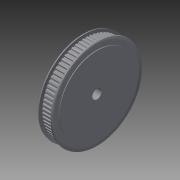
# Autodesk Inventor part: ATP72XL050-A-PUF_a
Saved by Autodesk Inventor 2014 SP2 (Build 180246200, 246)
## iProperties
Created: 2018-08-04
Part Number: ATP72XL050-A-PUF_a
Material: Generic
Catalog Web Link: www.cadenas.de
Description: ATP_ _XL025, ATP_ _XL031, ATP_ _ XL037, ATP_ _XL050, BTP_ _XL025, BTP_ _XL031, BTP_ _XL037, BTP_ _XL050, KTP_ _XL025, KTP_ _XL031, KTP_ _ XL037, KTP_ _XL050, NTP_ _XL025, NTP_ _XL031, NTP_ _ XL037, NTP_ _XL050, MTP_ _XL025, MTP_ _ XL037, MTP_ _XL050, MTPB_ _XL025, MTPB_ _ XL037, MTPB_ _XL050, MTPP_ _XL025, MTPP_ _ XL037, MTPP_ _XL050, STP_ _XL025, STP_ _ XL037, STP_ _XL050_aI-Timing Pulleys XL Type
Vendor: MISUMI
Document SubType Name: Modeling
Designer: psadmin
Manufacturer: MISUMI
Mass: 194.41 g
Surface Area: 364.949 cm^2
Volume: 194.41 cm^3
Density: 1 g/cm^3
Appearance: PSOLRGB-192-192-192
Category: PARTsolutions
Company: MISUMI
Title: ATP72XL050-A-PUF_a
Author: Cadenas PARTsolutions
Comments: Timing Pulleys XL Type
PSOL_IDENT_0: {$CADENAS_DATA\23d-libs\misumi\metric\51_timing_pulleys\timing_pulleys_inch\atp_xl_inch.prj},699 {VT
PSOL_IDENT_1: YP=3D},{NB=ATP72XL050-A-PUF_a},{LINA=ATP72XL050-A-PUF_a},{NN=ATP_ _XL025, ATP_ _XL031, ATP_ _ XL037,
PSOL_IDENT_2: ATP_ _XL050, BTP_ _XL025, BTP_ _XL031, BTP_ _XL037, BTP_ _XL050, KTP_ _XL025, KTP_ _XL031, KTP_ _ X
PSOL_IDENT_3: L037, KTP_ _XL050, NTP_ _XL025, NTP_ _XL031, NTP_ _ XL037, NTP_ _XL050, MTP_ _XL025, MTP_ _ XL037, M
PSOL_IDENT_4: TP_ _XL050, MTPB_ _XL025, MTPB_ _ XL037, MTPB_ _XL050, MTPP_ _XL025, MTPP_ _ XL037, MTPP_ _XL050, ST
PSOL_IDENT_5: P_ _XL025, STP_ _ XL037, STP_ _XL050_aI},{DATE=30.03.2018 07:26:26},{GEOMDATE=12.01.2011 12:59:00},{
PSOL_IDENT_6: VERSION=},{LINEID=280},{WBVAR=MATP,ST,TNW,PS,SHS,DD,ALT2,M,QSC,QFC,QTC,ALT7,K,KSC,KFC,KTC,ALT1,ALT3,
PSOL_IDENT_7: ALT4,ALT5,FC,ALT6,TPC,ALT8,BC,ALT9,SLH},{WBNUMERIC=DD,QSC,QFC,QTC,K,KSC,KFC,KTC,FC,TPC,BC,SLH}  {NB=
PSOL_IDENT_8: ATP72XL050-A-PUF_a},{LINA=ATP72XL050-A-PUF_a},{KT=DUMMY},{PN=ATP72XL050-A-PUF},{TYPE=ATP},{MATP=ATP}
PSOL_IDENT_9: ,{MATPA='ATP','2017 Aluminum Alloy (Duralumin)','MTP','1045 Carbon Steel'},{MATF=5052 Aluminum Alloy
PSOL_IDENT_10: },{ST=CA},{HARD=-},{STA= 'CA' , 'Clear Anodize' , 'BA','Black Anodize','HAT','Hard Clear Anodize','E
PSOL_IDENT_11: NP' , 'Electroless Nickel Plating' },{NT=72},{TNW=XL050},{TNW1=      'XL025','XL031','XL037','XL050'
PSOL_IDENT_12: },{BW=12.7mm (1/2inch)},{A=14.0},{W=19.0},{L=28},{PS=A},{PSA='A','B'},{S
PSOL_IDENT_13: HS=P},{SHS1= 'H','Inch Round Hole', 'P','Inch Round Hole + Tap','N','Inch ANSI Key Groove Hole'},{SH
PSOL_IDENT_14: S2=-PUF},{SHSA= 'H','Inch Round Hole', 'P','Inch Round Hole + Tap','N','Inch ANSI Key Groove Hole'},
PSOL_IDENT_15: {SHSB= 'H','Inch Round Hole', 'P','Inch Round Hole + Tap','N','Inch ANSI Key Groove Hole'},{DD=0.5},
PSOL_IDENT_16: {DDINCH=12.7},{DD1=0.5,0.625,0.75,0.875,1},{DDH=0.5,0.625,0.75,0.875,1,1.25,1.375,1.5,1.625,1.75,1.8
PSOL_IDENT_17: 75,2},{DDP=0.5,0.625,0.75,0.875,1},{DDN=0.5,0.625,0.75,0.875,1},{DDNK=10},{DDC=10,12,15,16,18,19,20}
PSOL_IDENT_18: ,{DDV=[10:80/1]},{DDF=[10:34/1]},{DDY=[10:75/1]},{DD635=13},{Z=0},{Z1=0},{ZQRMIN=15},{ZMAX=94},{ZA=0
PSOL_IDENT_19: },{ZB=0},{ZAB=},{J=0},{JA=0},{JMAX=17.0},{JAB=},{QRMAX=94},{Q=0},{Q1=0},{Q2=},{R=0},{R1=0},{R2=},{S=
PSOL_IDENT_20: 0},{S1=0},{S2=},{SMAX=8},{T=0},{T1=0},{T2=},{TMAX=8},{PD=116.43},{OD=115.92},{D=0},{DB=40},{F=123},{
PSOL_IDENT_21: E=102},{DE=102},{BJS9=0},{TTTI=0},{TTT=0},{AC=-},{NDM=4.000},{WL=19},{ALT2=},{ALT2A= '','w/o Side Ta
PSOL_IDENT_22: pped Hole','-QFC','with QFC (4 Side Tapped Holes)','-QTC','with QTC (3 Side Tapped Holes)'
PSOL_IDENT_23: },{QMIN=20},{QMAX=95},{M=-},{MA= '-' },{MAA=},{NDMALT=0.000},{QSC=0},{QSCA=0},{QSCAA=},{QFC=0},{
PSOL_IDENT_24: QFCA=0},{QFCAA=},{QTC=0},{QTCA=0},{QTCAA=},{QCMIN=17},{QCMAX=98},{QC=0},{ALT7=},{ALT7A=    '','w/o S
PSOL_IDENT_25: ide Through Hole','-KFC','with KFC (4 Side Through Holes)','-KTC','with KTC (3 Side Through Holes)'
PSOL_IDENT_26: },{ALT71=1},{ALT72=    '','w/o Side Through Hole','-KFC','with KFC (4 Side Through Holes)' },{ALT7
PSOL_IDENT_27: 3=    '','w/o Side Through Hole','-KTC','with KTC (3 Side Through Holes)' },{K=0.0},{KSC=0},{KSCA=
PSOL_IDENT_28: [0:0]       },{KSCAA=},{KFC=0},{KFCA=  [0:0]       },{KFCAA=},{KTC=0},{KTCA=  [0:0]       },{KTCAA=}
PSOL_IDENT_29: ,{KC=0},{KCMIN=17},{KCMAX=98},{KA=0},{KMAX=13.0},{KPN=},{ALT1=},{ALT1A='','w/o KC90 (Set Screw Angle
PSOL_IDENT_30: )','-KC90','with KC90 (Set Screw Angle)'},{ALT3=},{ALT4=},{ALT4A= '', 'w/o Flange Attached on One Si
PSOL_IDENT_31: de Only', '-RFC'  , 'with RFC (Flange Attached on The hub Side Only)', '-LFC'  , 'with LFC (Flange A
PSOL_IDENT_32: ttached on The Opposite Side Only)' },{ALT5=},{ALT5A='','w/o FC (Flange Cut)','-FC','with FC (Flange
PSOL_IDENT_33: Cut)'},{FC=0.0},{ODAINT=115},{FCMIN=118.0},{FCMAX=121.0},{FCA=0},{FCAA=},{ALFA=25},{ZUB=1.270},{TT=
PSOL_IDENT_34: 0.5},{TAP1=28.000},{TAP2=0.000},{TAP=0.000},{MM=2.5},{ALT6=},{ALT6A= '','w/o TPC (Tapped Hole Dimens
PSOL_IDENT_35: ion)','-TPC','with TPC (Tapped Hole Dimension)'},{TPC=0},{TPCA=           0,'N/A'         },{TPCAA=}
PSOL_IDENT_36: ,{ALT8=},{ALT8A=   '','N/A'                         },{BC=0.0},{BCCA=0},{BCCAMIN=7},{BCPLANE=9.5},{B
PSOL_IDENT_37: CCAMAX=9},{BCAA=},{TMP=},{KTT=52.11},{KYY=5.85},{PLANE=19},{TIF=1},{RUPE=2},{ALT9=},{ALT9A= '','w/o
PSOL_IDENT_38: SLH (Set Screw Length)','-SLH','with SLH (Set Screw Length)' },{SLH=0},{SLHA=0},{SLHPN=},{LS=3},{WS=
PSOL_IDENT_39: 4},{SL=57.96},{SL2=57.96},{ANG=120},{SCREWALG=1},{WLBC=19},{DDPN=F},{BBINCH=3.125}
NN: ATP_ _XL025, ATP_ _XL031, ATP_ _ XL037, ATP_ _XL050, BTP_ _XL025, BTP_ _XL031, BTP_ _XL037, BTP_ _XL050, KTP_ _XL025, KTP_ _XL031, KTP_ _ XL037, KTP_ _XL050, NTP_ _XL025, NTP_ _XL031, NTP_ _ XL037, NTP_ _XL050, MTP_ _XL025, MTP_ _ XL037, MTP_ _XL050, MTPB_ _XL025, MTPB_ _ XL037, MTPB_ _XL050, MTPP_ _XL025, MTPP_ _ XL037, MTPP_ _XL050, STP_ _XL025, STP_ _ XL037, STP_ _XL050_aI
NT: 72
NB: ATP72XL050-A-PUF_a
NBSYN: $PN._a
LINA: ATP72XL050-A-PUF_a
PN: ATP72XL050-A-PUF
MATP: 2017 Aluminum Alloy (Duralumin)
MATF: 5052 Aluminum Alloy
ST: Clear Anodize
HARD: -
TNW: XL050
BW: 12.7mm (1/2inch)
A: 14
W: 19
L: 28
PS: A
SHS: Inch Round Hole + Tap
DD: 0
PD: 116.43
OD: 115.92
D: 0
F: 123
E: 102
AC: -
ALT2: w/o Side Tapped Hole
M: -
QSC: 0
QFC: 0
QTC: 0
ALT7: w/o Side Through Hole
K: 0
KSC: 0
KFC: 0
KTC: 0
ALT1: w/o KC90 (Set Screw Angle)
ALT3: w/o NFC (Flange not Attached)
ALT4: w/o Flange Attached on One Side Only
ALT5: w/o FC (Flange Cut)
FC: 0
ALT6: w/o TPC (Tapped Hole Dimension)
TPC: 0
ALT8: N/A
BC: 0
ALT9: w/o SLH (Set Screw Length)
SLH: 0
SUPPLIER: MISUMI
ARTICLENO: ATP72XL050-A-PUF_a
BOMINFO: ATP72XL050-A-PUF_a
CREATOR: CADENAS GmbH
Autodesk Inventor part; units mm, degrees
ref_plane "YZ Plane" through (0, 0, 0) normal (1, 0, 0) x (0, 1, 0)
ref_plane "XZ Plane" through (0, 0, 0) normal (0, 1, 0) x (-1, 0, 0)
ref_plane "XY Plane" through (0, 0, 0) normal (0, 0, 1) x (1, 0, 0)
sketch "Sketch_5" plane through (0, 0, 0) normal (0, 0, 1) x (1, 0, 0)
  line L0 (28, 0) -> (0, 0)
  line L1 (0, 6.35) -> (19, 6.35)
  line L2 (19, 6.35) -> (19, 51)
  line L3 (19, 51) -> (18.1, 51)
  line L4 (18.1, 51) -> (18.1, 57.9998)
  line L5 (18.1, 57.9998) -> (18.9431, 61.0772)
  line L6 (18.9431, 61.0772) -> (17.4, 61.5)
  line L7 (17.4, 61.5) -> (16.5, 58.215)
  line L8 (16.5, 58.215) -> (16.5, 57.96)
  line L9 (16.5, 57.96) -> (2.5, 57.96)
  line L10 (2.5, 57.96) -> (2.5, 58.215)
  line L11 (2.5, 58.215) -> (1.6, 61.5)
  line L12 (1.6, 61.5) -> (0.0569, 61.0772)
  line L13 (0.0569, 61.0772) -> (0.9, 57.9998)
  line L14 (0.9, 57.9998) -> (0.9, 51)
  line L15 (0.9, 51) -> (0, 51)
  line L16 (0, 51) -> (0, 6.35)
  constraints: 34 end point
revolve "Revolution1" add sketch "Sketch_5" angle 360 about axis through (28, 0, 0) along (1, 0, 0)
sketch "Sketch_2" plane through (2.5, 0, 0) normal (1, 0, 0) x (0, 0, -1)
  line L0 (-1.6845, 77.28) -> (-1.6845, 57.9355)
  arc A0 (-1.114, 57.5836) -> (-1.6845, 57.9355) centre (-1.6668, 57.3258) ccw
  line L1 (-1.114, 57.5836) -> (-0.8006, 56.9117)
  arc A1 (-0.8006, 56.9117) -> (-0.2452, 56.5595) centre (-0.2478, 57.1695) ccw
  arc A2 (0.2452, 56.5595) -> (-0.2452, 56.5595) centre (0, 0) ccw
  arc A3 (0.2452, 56.5595) -> (0.8006, 56.9117) centre (0.2478, 57.1695) ccw
  line L2 (0.8006, 56.9117) -> (1.114, 57.5836)
  arc A4 (1.6845, 57.9355) -> (1.114, 57.5836) centre (1.6668, 57.3258) ccw
  line L3 (1.6845, 57.9355) -> (1.6845, 77.28)
  line L4 (1.6845, 77.28) -> (-1.6845, 77.28)
  constraints: 10 end point, 10 point on circle, 5 centre point
extrude "Extrusion1" cut sketch "Sketch_2" along normal blind 14
pattern_circular "Circular Pattern1" count 72 over 360 about axis through (2.5, 0, 0) along (1, 0, 0) of "Extrusion1"
sketch "Sketch_21" plane through (9.5, 0, 0) normal (1, 0, 0) x (0, 0, -1)
  line L0 (0, 0) -> (0, 57.96)
  line L1 (0, 57.96) -> (1.621, 57.96)
  line L2 (1.621, 57.96) -> (1.621, 0)
  line L3 (1.621, 0) -> (0, 0)
  line L4 (0, 0) -> (0, 57.96)
  constraints: 10 end point
revolve "Revolution2" cut sketch "Sketch_21" angle 360 about axis through (9.5, 0, 0) along (0, -1, 0)
thread "Thread1" size "M4x0.7" class "6H" standard "ISO Metric profile" length 51.61
sketch "Sketch_22" plane through (9.5, 0, 0) normal (1, 0, 0) x (0, 0, -1)
  line L0 (0, 0) -> (50.1948, -28.98)
  line L1 (50.1948, -28.98) -> (49.3843, -30.3838)
  line L2 (49.3843, -30.3838) -> (-0.8105, -1.4038)
  line L3 (-0.8105, -1.4038) -> (0, 0)
  line L4 (0, 0) -> (50.1948, -28.98)
  constraints: 10 end point
revolve "Revolution3" cut sketch "Sketch_22" angle 360 about axis through (9.5, 0, 0) along (0, 0.5, 0.8660254)
thread "Thread2" size "M4x0.7" class "6H" standard "ISO Metric profile" full length
ref_plane "to_s1_XY" through (9.5, 57.96, 0) normal (0, 1, 0) x (1, 0, 0)
ref_plane "to_s1_YZ" through (9.5, 57.96, 0) normal (1, 0, 0) x (0, 0, -1)
ref_plane "to_s1_ZX" through (9.5, 57.96, 0) normal (0, 0, -1) x (0, 1, 0)
ref_plane "to_s2_XY" through (9.5, -28.98, -50.1948) normal (0, -0.5, -0.8660254) x (1, 0, 0)
ref_plane "to_s2_YZ" through (9.5, -28.98, -50.1948) normal (1, 0, 0) x (0, -0.8660254, 0.5)
ref_plane "to_s2_ZX" through (9.5, -28.98, -50.1948) normal (0, -0.8660254, 0.5) x (0, -0.5, -0.8660254)
body "Solid1"
